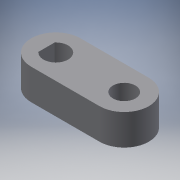
# Autodesk Inventor part: crank
Saved by Autodesk Inventor 2017 (Build 210142000, 142)
## iProperties
Created: 2018-01-02
Part Number: crank
Material: Generic
Document SubType Name: Modeling
Designer: RLanting
Density: 1 g/cm^3
Appearance: Default
Author: RLanting
Autodesk Inventor part; units mm, degrees
ref_plane "YZ Plane" through (0, 0, 0) normal (1, 0, 0) x (0, 1, 0)
ref_plane "XZ Plane" through (0, 0, 0) normal (0, 1, 0) x (-1, 0, 0)
ref_plane "XY Plane" through (0, 0, 0) normal (0, 0, 1) x (1, 0, 0)
sketch "Sketch1" plane through (0, 0, 0) normal (0, 0, 1) x (1, 0, 0)
  line L0 (0, 0) -> (22.225, 0) construction
  line L1 (0, -8) -> (22.225, -8)
  line L2 (22.225, 8) -> (0, 8)
  arc A0 (0, 8) -> (0, -8) centre (0, 0) ccw
  arc A1 (22.225, -8) -> (22.225, 8) centre (22.225, 0) ccw
  circle A2 centre (22.225, 0) radius 3.65
  circle A3 centre (0, 0) radius 4
  point P0 (11.1125, 0)
  dimension "d0" = 22.225
  dimension "d1" = 8
  dimension "d2" = 7.3
  dimension "d3" = 16
  constraints: 8 end point, 4 centre point, 4 point on circle, 4 tangent, 2 coincident, 1 horizontal, 1 midpoint, 1 parallel
  measures "d0" distance of L0.start L0.end
  measures "d1" diameter of A3
  measures "d2" diameter of A2
  measures "d3" distance between parallel lines of L1 L2
extrude "Extrusion1" add sketch "Sketch1" along normal blind 10
sketch "Sketch2" plane through (0, 0, 10) normal (0, 0, 1) x (1, 0, 0)
  circle A0 centre (0, 0) radius 4 projected
  arc A1 (-3, 2.6458) -> (-3, -2.6458) centre (0, 0) ccw
  line L0 (-3, 2.6458) -> (-3, -2.6458)
  dimension "d6" = 7
  constraints: 2 end point, 2 point on circle, 1 centre point, 1 coincident, 1 vertical, 2 other
extrude "Extrusion2" add sketch "Sketch2" against normal up to surface (10 mm away) contours L0 A0 picked at (-3.1815, -0.6179)
body "Solid1"
